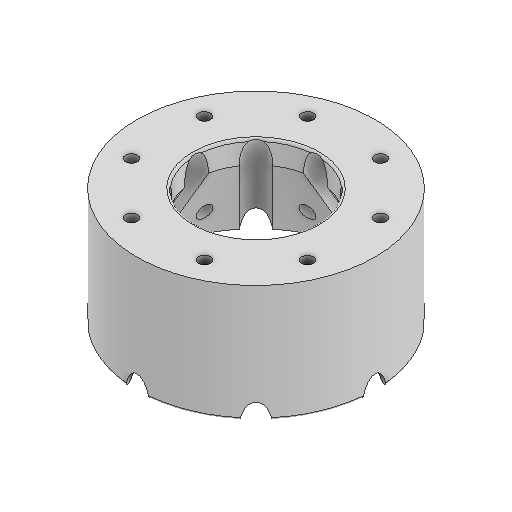
# Autodesk Inventor part: 3DP_ASA_Bottom_Cone_Top_Half
Saved by Autodesk Inventor 2026.1 (Build 301233000, 233)
## iProperties
Created: 2025-06-19
Part Number: 3DP_ASA_Bottom_Cone_Top_Half
Material: Generic
Document SubType Name: Modeling
Designer: User
Density: 1 g/cm^3
Appearance: Default
Author: User
Autodesk Inventor part; units mm, degrees
ref_plane "YZ Plane" through (0, 0, 0) normal (1, 0, 0) x (0, 1, 0)
ref_plane "XZ Plane" through (0, 0, 0) normal (0, 1, 0) x (-1, 0, 0)
sketch "Sketch1" plane through (0, 0, 0) normal (0, 0, 1) x (1, 0, 0)
  line L0 (0, 53.9615) -> (-20, 53.9615)
  line L1 (-20, 53.9615) -> (-50, 2)
  line L2 (-50, 2) -> (-50, 0)
  line L3 (-50, 0) -> (0, 0)
  line L4 (0, 0) -> (0, 53.9615)
  line L5 (0, -10.7923) -> (0, 64.7538) projected
  line L6 (-50, 2) -> (-50, 53.9615)
  line L7 (-50, 53.9615) -> (-20, 53.9615)
  dimension "d0" = 50
  dimension "d2" = 20
  dimension "d3" = 30
  dimension "d4" = 2
  dimension "d5" = 53.9615
  constraints: 14 end point, 3 perpendicular, 2 vertical, 1 horizontal
  measures "d0" distance between parallel lines of L4 L2
  measures "d2" distance of L0.start L0.end
  measures "d3" angle of L4 L1
  measures "d4" distance of L1.end L2.end
  measures "d5" distance between parallel lines of L3 L0
revolve "Revolution1" add sketch "Sketch1" angle 360 about axis through (0, -10, 0) along (0, 1, 0) contours L1 L6 L7
sketch "Sketch6" plane through (0, 53.9615, 0) normal (0, 1, 0) x (1, 0, 0)
  circle A0 centre (0, 0) radius 50 projected
  circle A1 centre (0, 0) radius 20 projected
  line L0 (15.2271, -20) -> (-17.6314, -20)
  dimension "d37" = 20
  constraints: 2 end point, 1 horizontal
  measures "d37" distance from line of point (0, 0) L0
ref_plane "Work Plane2" through (15.2271, 53.9615, 20) normal (0, 0.866, -0.5) x (-1, 0, 0)
sketch "Sketch7" plane through (15.2271, 53.9615, 20) normal (0, 0.866, -0.5) x (-1, 0, 0)
  ellipse E0 centre (15.2271, -17.3205) end of major axis (-34.7729, -17.3205) minor radius 43.3013 projected
  ellipse E1 centre (15.2271, -17.3205) end of major axis (-4.7729, -17.3205) minor radius 17.3205 projected
  circle A0 centre (15.2271, -0.25) radius 5
  point P0 (15.2271, -44.3013)
  point P1 (15.2271, 0)
  dimension "d39" = 0.25
  dimension "d40" = 10
  constraints: 1 centre point, 1 coincident, 1 vertical alignment, 2 other
  measures "d39" distance of point (15.227, 0) point (15.227, -0.25)
  measures "d40" diameter of A0
extrude "Extrusion2" cut sketch "Sketch7" along normal through all both and the other way through all contours A0 E1 | E1 A0 picked at (15.4204, -1.7795) picked at (15.3824, 1.5353)
pattern_circular "Circular Pattern3" count 8 over 360 about axis through (0, -10, 0) along (0, 1, 0) of "Extrusion2"
sketch "Sketch8" plane through (0, 53.9615, 0) normal (0, 1, 0) x (1, 0, 0)
  line L0 (0, 0) -> (-15.3073, -36.9552)
  line L1 (0, 0) -> (0, -50)
  circle A0 centre (0, 0) radius 50 projected
  dimension "d46" = 40
  dimension "d47" = 22.5
  constraints: 4 end point, 1 coincident, 1 vertical, 1 vertical alignment, 1 other
  measures "d46" distance of L0.start L0.end
  measures "d47" angle of L1 L0
hole "Hole3" at (-15.3073, 53.9615, 36.9552) direction (0, -1, 0) diameter 5 end through all
pattern_circular "Circular Pattern4" count 8 over 360 about axis through (0, -10, 0) along (0, 1, 0) of "Hole3"
sketch "Sketch9" plane through (0, 53.9615, 0) normal (0, 1, 0) x (1, 0, 0)
  circle A0 centre (0, 0) radius 25.5
  dimension "d58" = 51
  constraints: 1 centre point, 1 coincident
  measures "d58" diameter of A0
extrude "Extrusion3" cut sketch "Sketch9" against normal through all
fillet "Fillet1" radius 1 8 edges at (46.194, 2, 19.1342) (46.194, 2, -19.1342) (19.1342, 2, -46.194) (-19.1342, 2, -46.194) (-46.194, 2, -19.1342) (-46.194, 2, 19.1342) (-19.1342, 2, 46.194) (19.1342, 2, 46.194)
fillet "Fillet2" radius 1 1 edges at (-25.5, 53.9615, 0)
body "Solid1"
